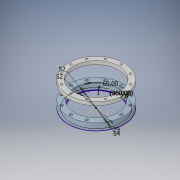
# Autodesk Inventor part: Enclosure
Saved by Autodesk Inventor 2018.3 (Build 223284000, 284)
## iProperties
Created: 2018-07-23
Part Number: Enclosure
Material: Generisch
Document SubType Name: Modeling
Designer: JochenAlt
Density: 1 g/cm^3
Appearance: Vorgabe
Author: JochenAlt
Autodesk Inventor part; units mm, degrees
ref_plane "YZ Plane" through (0, 0, 0) normal (1, 0, 0) x (0, 1, 0)
ref_plane "XZ Plane" through (0, 0, 0) normal (0, 1, 0) x (-1, 0, 0)
sketch "Skizze1" plane through (0, 0, 0) normal (0, 0, 1) x (1, 0, 0)
  circle A0 centre (0, 0) radius 29 construction
  line L0 (0, 44.8) -> (0, -44.8) construction
  line L1 (-44.8, 0) -> (44.8, 0) construction
  line L2 (0, 0) -> (-28.9685, 16.725) construction
  circle A1 centre (0, 29) radius 1.6
  circle A2 centre (-14.5, 25.1147) radius 1.6
  circle A3 centre (-25.1147, 14.5) radius 1.6
  circle A4 centre (-29, 0) radius 1.6
  circle A5 centre (-25.1147, -14.5) radius 1.6
  circle A6 centre (-14.5, -25.1147) radius 1.6
  circle A7 centre (0, -29) radius 1.6
  circle A8 centre (14.5, -25.1147) radius 1.6
  circle A9 centre (25.1147, -14.5) radius 1.6
  circle A10 centre (29, 0) radius 1.6
  circle A11 centre (25.1147, 14.5) radius 1.6
  circle A12 centre (0, 0) radius 32
  circle A13 centre (14.5, 25.1147) radius 1.6
  circle A14 centre (0, 0) radius 26
  circle A15 centre (0, 0) radius 26
  circle A16 centre (0, 0) radius 25
  circle A17 centre (0, 29) radius 1.2
  circle A18 centre (-14.5, 25.1147) radius 1.2
  circle A19 centre (-25.1147, 14.5) radius 1.2
  circle A20 centre (-29, 0) radius 1.2
  circle A21 centre (-25.1147, -14.5) radius 1.2
  circle A22 centre (-14.5, -25.1147) radius 1.2
  circle A23 centre (0, -29) radius 1.2
  circle A24 centre (14.5, -25.1147) radius 1.2
  circle A25 centre (25.1147, -14.5) radius 1.2
  circle A26 centre (29, 0) radius 1.2
  circle A27 centre (25.1147, 14.5) radius 1.2
  circle A28 centre (14.5, 25.1147) radius 1.2
  circle A29 centre (0, 29) radius 2.5
  circle A30 centre (-14.5, 25.1147) radius 2.5
  circle A31 centre (-25.1147, 14.5) radius 2.5
  circle A32 centre (-29, 0) radius 2.5
  circle A33 centre (-25.1147, -14.5) radius 2.5
  circle A34 centre (-14.5, -25.1147) radius 2.5
  circle A35 centre (0, -29) radius 2.5
  circle A36 centre (14.5, -25.1147) radius 2.5
  circle A37 centre (25.1147, -14.5) radius 2.5
  circle A38 centre (29, 0) radius 2.5
  circle A39 centre (25.1147, 14.5) radius 2.5
  circle A40 centre (14.5, 25.1147) radius 2.5
  dimension "d1" = 29
  dimension "d17" = 60
  dimension "d32" = 360
  dimension "d107" = 64
  dimension "d111" = 52
  dimension "d112" = 52
  dimension "d113" = 1
  dimension "d120" = 2.4
  dimension "d123" = 360
  dimension "d127" = 3.2
  dimension "d128" = 5
  dimension "d131" = 360
  constraints: 40 centre point, 6 coincident, 2 concentric, 2 end point, 1 midpoint, 1 point on line, 1 vertical alignment, 89 other
  measures "d17" angle of L0 L2
  measures "d107" diameter of A12
  measures "d111" diameter of A14
  measures "d112" diameter of A15
  measures "d113" radial gap between concentric circles of A16 A14
  measures "d120" diameter of A17
  measures "d127" diameter of A1
  measures "d128" diameter of A29
extrude "Extrusion1" add sketch "Skizze1" along normal blind 2 contours A12
extrude "Extrusion2" add sketch "Skizze1" along normal blind 1.5 from surface at 2 contours A1 | A2 | A3 | A4 | A5 | A6 | A7 | A8 | A9 | A10 | A11 | A12 | A13 | A29 | A30 | A31 | A32 | A33 | A34 | A35 | A36 | A37 | A38 | A39 | A40
extrude "Extrusion25" add sketch "Skizze1" along normal blind 3.5 from surface at 3.5 contours A12 | A29 | A30 | A31 | A32 | A33 | A34 | A35 | A36 | A37 | A38 | A39 | A40
extrude "Extrusion24" add sketch "Skizze1" along normal blind 1 from surface at 7 contours A12 | A14 | A29 | A30 | A31 | A32 | A33 | A34 | A35 | A36 | A37 | A38 | A39 | A40
ref_plane "Arbeitsebene1" through (0, 0, 25) normal (0, 0, 1) x (1, 0, 0)
extrude "Extrusion20" add sketch "Skizze1" along normal blind 2 from surface at 25 separate body contours A12 | A29 | A30 | A31 | A32 | A33 | A34 | A35 | A36 | A37 | A38 | A39 | A40
extrude "Extrusion21" add sketch "Skizze1" along normal blind 2 from surface at 27 contours A1 | A2 | A3 | A4 | A5 | A6 | A7 | A8 | A9 | A10 | A11 | A12 | A13 | A29 | A30 | A31 | A32 | A33 | A34 | A35 | A36 | A37 | A38 | A39 | A40 bodies 2
